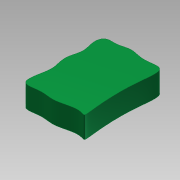
# Autodesk Inventor part: SOIC-10 micro (RM-10) board
Saved by Autodesk Inventor 2011 (Build 150239000, 239)
## iProperties
Created: 2010-12-28
Part Number: SOIC-10 micro (RM-10) board
Document SubType Name: Modeling
Designer: abbath
Density: 1 g/cm^3
Mass: 0.0326206 g
Surface Area: 0.72682 cm^2
Volume: 0.0326206 cm^3
Author: abbath
Autodesk Inventor part; units mm, degrees
ref_plane "YZ Plane" through (0, 0, 0) normal (1, 0, 0) x (0, 1, 0)
ref_plane "XZ Plane" through (0, 0, 0) normal (0, 1, 0) x (-1, 0, 0)
ref_plane "XY Plane" through (0, 0, 0) normal (0, 0, 1) x (1, 0, 0)
ref_plane "РабПлоскость3" through (0, 0, 0) normal (0, 0, 1) x (1, 0, 0)
sketch "Эскиз4" plane through (0, 0, 0) normal (0, 0, 1) x (1, 0, 0)
  spline S0 degree 5 poles (-1.0062, -0.2579) (-0.8885, -0.3986) (-0.5323, -0.4308) (0.3997, -0.0211) (0.8291, -0.8625) (3.0121, 0.5877) (3.236, -1.3184) (2.6612, 2.2671) (3.029, 4.4558) (3.1954, 5.8238) (1.6481, 4.8065) (0.7524, 5.7458) (-0.1167, 4.908) (-0.8665, 5.5075) (-1.307, 4.5266) (-0.5959, 3.5937) (-1.258, 2.8981) (-0.99, 1.8388) (-0.765, 1.468) (-1.1497, 0.3175) (-1.1253, -0.1155) (-1.0062, -0.2579) knots 0 0 0 0 0 0 0.072714 0.118006 0.178422 0.249496 0.31604 0.379743 0.448363 0.512581 0.564268 0.616427 0.668211 0.718882 0.76946 0.822531 0.880264 0.926431 1 1 1 1 1 1
  point P0 (0, 0)
  point P1 (1.0511, -0.3464)
  point P2 (2.6452, -0.1216)
  point P3 (2.9926, -0.1966)
  point P4 (2.8972, 1.4861)
  point P5 (2.9926, 4.8786)
  point P6 (2.7065, 5.2874)
  point P7 (1.6574, 5.2329)
  point P8 (0.6287, 5.3623)
  point P9 (-0.2024, 5.1988)
  point P10 (-0.7882, 5.1511)
  point P11 (-1.0539, 4.6606)
  point P12 (-0.9041, 3.6865)
  point P13 (-1.0539, 2.8486)
  point P14 (-1.0062, 2.0174)
  point P15 (-0.9585, 1.0569)
  constraints: 17 other
extrude "Выдавливание4" add sketch "Эскиз4" along normal blind 1.5
